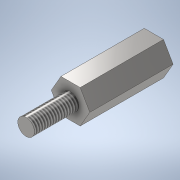
# Autodesk Inventor part: Spacer_M3_L15
Saved by Autodesk Inventor 2022 (Build 260153000, 153)
## iProperties
Created: 2022-02-05
Part Number: Spacer_M3_L15
Material: 鋼、合金
Document SubType Name: Modeling
Designer: satot
Density: 7.73 g/cm^3
Appearance: 半つや出し
Author: satot
Autodesk Inventor part; units mm, degrees
ref_plane "YZ Plane" through (0, 0, 0) normal (1, 0, 0) x (0, 1, 0)
ref_plane "XZ Plane" through (0, 0, 0) normal (0, 1, 0) x (-1, 0, 0)
ref_plane "XY Plane" through (0, 0, 0) normal (0, 0, 1) x (1, 0, 0)
sketch "スケッチ1" plane through (0, 0, 0) normal (1, 0, 0) x (0, 1, 0)
  line L0 (1.7321, -3) -> (-1.7321, -3)
  line L1 (-1.7321, -3) -> (-3.4641, 0)
  line L2 (-3.4641, 0) -> (-1.7321, 3)
  line L3 (-1.7321, 3) -> (1.7321, 3)
  line L4 (1.7321, 3) -> (3.4641, 0)
  line L5 (3.4641, 0) -> (1.7321, -3)
  point P0 (0, 0)
  point P1 (0, 0)
  dimension "d0" = 6
  constraints: 12 end point, 1 coincident, 1 horizontal alignment, 13 other
  measures "d0" distance between parallel lines of L3 L0
extrude "押し出し1" add sketch "スケッチ1" along normal blind 15
sketch "スケッチ2" plane through (15, 0, 0) normal (1, 0, 0) x (0, 0, -1)
  circle A0 centre (0, 0) radius 1.5
  dimension "d3" = 3
  constraints: 1 centre point, 1 coincident
  measures "d3" diameter of A0
extrude "押し出し2" add sketch "スケッチ2" along normal blind 8
thread "ねじ1" size "M3x0.5" class "6g" standard "ANSI Metric M Profile" full length
sketch "スケッチ3" plane through (0, 0, 0) normal (-1, 0, 0) x (0, 0, 1)
  point P0 (0, 0)
  point P1 (0, 0)
  constraints: 1 coincident
hole "穴1" at (0, 0, 0) direction (1, 0, 0) diameter 2.459 depth 10 tip angle 118 thread size "M3x0.5" class "6H" standard "ISO Metric profile"
